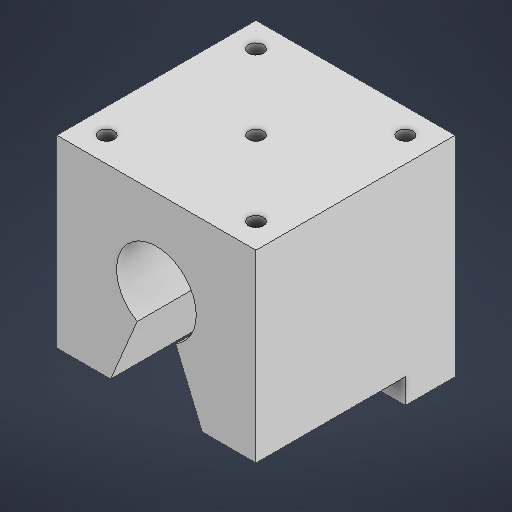
# Autodesk Inventor part: X Axis End
Saved by Autodesk Inventor 2025.1 (Build 291241000, 241)
## iProperties
Created: 2024-11-25
Part Number: X Axis End
Material: Generic
Document SubType Name: Modeling
Designer: jerem
Density: 1 g/cm^3
Appearance: Default
Author: jerem
Autodesk Inventor part; units mm, degrees
ref_plane "YZ Plane" through (0, 0, 0) normal (1, 0, 0) x (0, 1, 0)
ref_plane "XZ Plane" through (0, 0, 0) normal (0, 1, 0) x (-1, 0, 0)
ref_plane "XY Plane" through (0, 0, 0) normal (0, 0, 1) x (1, 0, 0)
sketch "Sketch1" plane through (0, 0, 0) normal (0, 0, 1) x (1, 0, 0)
  circle A0 centre (0, 24.7) radius 8
  line L0 (0, 24.7) -> (0, 0) construction
  line L1 (0, 0) -> (-20, 0) construction
  line L2 (-20, 0) -> (-20, 5) construction
  line L3 (-20, 5) -> (-9.2, 5) construction
  line L4 (-9.2, 5) -> (-3.85, 17.6873)
  line L5 (0, 0) -> (20, 0) construction
  line L6 (20, 0) -> (20, 5) construction
  line L7 (20, 5) -> (9.2, 5) construction
  line L8 (9.2, 5) -> (3.85, 17.6873)
  line L9 (0, 24.7) -> (0, 32.7) construction
  line L10 (-3.85, 17.6873) -> (3.85, 17.6873) construction
  line L11 (-8.85, 0) -> (-4.5, 5.6) construction
  line L12 (-4.5, 5.6) -> (0, 5.6) construction
  line L13 (0, 5.6) -> (4.5, 5.6) construction
  line L14 (4.5, 5.6) -> (8.85, 0) construction
  line L15 (-20, 5) -> (-20, 42)
  line L16 (-20, 42) -> (20, 42)
  line L17 (20, 42) -> (20, 5)
  line L18 (-20, 5) -> (20, 5)
  line L19 (20, 5) -> (-20, 5)
  line L20 (-20, 5) -> (-20, 0)
  line L21 (-20, 0) -> (20, 0)
  line L22 (20, 0) -> (20, 5)
  point P0 (0, 42)
  point P1 (-9.2, 5)
  point P2 (9.2, 5)
  dimension "d0" = 16
  dimension "d1" = 40
  dimension "d2" = 5
  dimension "d3" = 10.8
  dimension "d4" = 32.7
  dimension "d5" = 7.7
  dimension "d6" = 9
  dimension "d7" = 5.6
  dimension "d8" = 17.7
  dimension "d91" = 42
  constraints: 46 end point, 8 perpendicular, 6 equal length, 5 horizontal, 3 point on circle, 3 point on line, 3 vertical, 2 coincident, 2 parallel, 1 centre point, 1 midpoint
  measures "d0" diameter of A0
  measures "d1" distance between parallel lines of L6 L2
  measures "d2" distance of L1.end L3.start
  measures "d3" distance of L3.start L4.start
  measures "d4" distance of L5.start L9.end
  measures "d5" distance of L10.start L8.end
  measures "d6" distance of L14.start L12.start
  measures "d7" distance between parallel lines of L1 L12
  measures "d8" distance of L14.end L11.start
  measures "d91" distance between parallel lines of L1 L16
extrude "Extrusion1" add sketch "Sketch1" along normal blind 30 contours A0 L4 L18 L15 L16 L17 L8
extrude "Extrusion2" add sketch "Sketch1" against normal blind 10
sketch "Sketch6" plane through (-20, 42, 30) normal (0, 1, 0) x (1, 0, 0)
  line L0 (0, 40) -> (0, 0) projected
  line L1 (40, 0) -> (0, 0) projected
  line L2 (40, 0) -> (40, 40) projected
  line L3 (0, 40) -> (40, 40) projected
  line L4 (0, 40) -> (40, 0) construction
  line L5 (40, 40) -> (0, 0) construction
  circle A0 centre (35, 5) radius 1.5
  circle A1 centre (5, 5) radius 1.5
  circle A2 centre (5, 35) radius 1.5
  circle A3 centre (35, 35) radius 1.5
  line L6 (35, 35) -> (35, 5) construction
  line L7 (5, 5) -> (35, 5) construction
  line L8 (5, 5) -> (5, 35) construction
  circle A4 centre (20, 20) radius 1.5
  point P0 (20, 30)
  dimension "d69" = 30
  dimension "d70" = 3
  dimension "d73" = 3
  constraints: 10 end point, 5 centre point, 4 point on line, 3 equal radius, 3 perpendicular, 2 midpoint, 1 coincident
  measures "d69" distance of L8.start L7.end
  measures "d70" diameter of A0
  measures "d73" diameter of A4
extrude "Extrusion8" cut sketch "Sketch6" against normal blind 5 contours A0 | A1 | A2 | A3
extrude "Extrusion9" cut sketch "Sketch6" against normal through all contours A4
sketch "Sketch7" plane through (-20, 5, 30) normal (-1, 0, 0) x (0, 0, 1)
  line L0 (-30, 0) -> (0, 0) projected
  line L1 (0, 37) -> (0, 0) projected
  line L2 (-40, 37) -> (0, 37) projected
  line L3 (-40, -5) -> (-40, 37) projected
  line L4 (-30, -5) -> (-40, -5) projected
  line L5 (-30, 0) -> (-30, -5) projected
  line L6 (-40, 16) -> (-20, 16) construction
  circle A0 centre (-20, 16) radius 1.5
  point P0 (-30, -5)
  dimension "d92" = 3
  constraints: 2 end point, 1 centre point, 1 coincident, 1 horizontal, 1 midpoint
  measures "d92" diameter of A0
extrude "Extrusion11" cut sketch "Sketch7" against normal blind 5 contours A0
body "Solid1"
